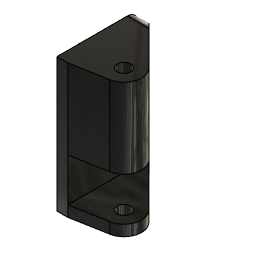
3030 Idler Bracket B Front_1X v4 (Autodesk Fusion 360 design; units mm, degrees)
Autodesk Fusion 360 part; units mm, degrees
sketch "Sketch1" plane through (0, 0, 0) normal (1, 0, 0) x (0, 1, 0)
  line L0 (0, 16) -> (20, 16)
  line L1 (20, 16) -> (20, 0)
  line L2 (20, 0) -> (0, 0)
  line L3 (0, 0) -> (0, 16)
  dimension "d2462_1" = 20
  dimension "d2463_1" = 16
  constraint horizontal L0
  constraint vertical L1
  constraint horizontal L2
  constraint vertical L3
  constraint coincident L2.end L3.start
  measures "d2462_1" distance of L0.start L0.end
  measures "d2463_1" distance of L0.start L2.end
extrude "Extrude1" add sketch "Sketch1" along normal blind 4
sketch "Sketch2" plane through (0, 0, 16) normal (0, 0, 1) x (-1, 0, 0)
  line L0 (0, -20) -> (0, 0)
  line L1 (0, 0) -> (-4, 0)
  line L2 (-4, 0) -> (-4, -20)
  line L3 (-4, -20) -> (0, -20)
  line L4 (-4, -10) -> (-29.8619, -10) construction
  circle A0 centre (-16, -21.24) radius 6 construction
  circle A1 centre (-42.1729, -8.5) radius 6.11 construction
  line L5 (-16, -15.24) -> (-27.2824, -15.24) construction
  line L6 (-42.1729, -14.61) -> (-27.2824, -14.61) construction
  line L7 (-27.2824, -15.24) -> (-27.2824, -14.61) construction
  line L8 (-16, -15.24) -> (-16, -13.84) construction
  line L9 (-16, -13.84) -> (-48.5157, -13.84) construction
  circle A2 centre (-16, -21.24) radius 2.5
  arc A3 (-20.6028, -16.6504) -> (-11.9535, -26.3269) centre (-16, -21.24) ccw
  line L10 (-4, -20) -> (-11.9535, -26.3269)
  line L11 (-4, 0) -> (-20.6028, -16.6504)
  dimension "d4861_1" = 12
  dimension "d4864_1" = 12
  dimension "d4867_1" = 12.22
  dimension "d4871_1" = 0.63
  dimension "d4872_1" = 1.4
  dimension "d4873_1" = 0.77
  dimension "d4874_1" = 5
  dimension "d4876_1" = 4
  dimension "d5002" = 8.5
  constraint midpoint L2 L4.start
  constraint perpendicular L2 L4
  constraint coincident A0 L5.start
  constraint tangent A0 L5
  constraint parallel L4 L5
  constraint coincident A1 L6.start
  constraint horizontal L6
  constraint perpendicular L5 L7
  constraint coincident L6.end L7.end
  constraint tangent A1 L6
  constraint perpendicular L5 L8
  constraint perpendicular L8 L9
  constraint concentric A0 A2
  constraint concentric A2 A3
  constraint coincident L2.end L3.start
  constraint coincident L1.end L2.start
  constraint tangent A3 L10
  constraint tangent A3 L11
  measures "d4861_1" diameter of A0
  measures "d4864_1" distance of L2 A0.centre
  measures "d4867_1" diameter of A1
  measures "d4871_1" distance of L5.end L6.end
  measures "d4872_1" distance of L5 L9
  measures "d4873_1" distance of A1 L9
  measures "d4874_1" diameter of A2
  measures "d4876_1" distance of A2 A3
  measures "d5002" distance of L1 A1.centre
extrude "Extrude2" add sketch "Sketch2" along normal blind 4
extrude "Extrude3" add sketch "Sketch2" against normal blind 4 from surface at -16
extrude "Extrude6" add 1 faces at (1.3333, 20, 10.6667) along direction (0, 1, 0) blind 10
sketch "Sketch5" plane through (0, 0, 20) normal (0, 0, 1) x (-1, 0, 0)
  line L0 (0, -30) -> (0, 0)
  line L1 (0, 0) -> (-4, 0)
  line L2 (-4, -20) -> (-4, -30)
  line L3 (-4, -30) -> (0, -30)
  line L4 (-4, -30) -> (0, -30)
  line L5 (0, 0) -> (0, -30)
  line L6 (-4, -20) -> (-4, -30)
  line L7 (-4, 0) -> (0, 0)
  line L8 (-4, -30) -> (-17.1494, -27.6376)
  circle A0 centre (-16, -21.24) radius 2.5
  line L9 (-4, 0) -> (-20.6028, -16.6504)
  arc A1 (-20.6028, -16.6504) -> (-11.9535, -26.3269) centre (-16, -21.24) ccw
  line L10 (-11.9535, -26.3269) -> (-4, -20)
  circle A2 centre (-16, -21.24) radius 2.5
  line L11 (-20.6028, -16.6504) -> (-4, 0)
  arc A3 (-20.6028, -16.6504) -> (-11.9535, -26.3269) centre (-16, -21.24) ccw
  line L12 (-4, -20) -> (-11.9535, -26.3269)
  constraint coincident L6 L2.end
  constraint coincident L8.end A3
  constraint tangent L8 A3
  constraint coincident L2.end L3.start
extrude "Extrude7" add sketch "Sketch5" against normal up to surface (4 mm away) contours L2 L6 L8 A1 L10 A3 L12
extrude "Extrude8" add sketch "Sketch5" along normal up to surface (4 mm away) from surface at -24 contours L2 L6 L8 A1 L10 A3 L12
sketch "Sketch4" plane through (4, 0, 0) normal (1, 0, 0) x (0, 1, 0)
  line L0 (0, 0) -> (30, 0)
  line L1 (30, 16) -> (0, 16)
  line L2 (30, -4) -> (0, -4)
  line L3 (0, 20) -> (30, 20)
  line L4 (0, 8) -> (10, 8)
  line L5 (30, 8) -> (15, 8)
  line L6 (30, 0) -> (30, 16)
  line L7 (0, 16) -> (0, 0)
  line L8 (0, -4) -> (0, 20)
  line L9 (30, 20) -> (30, -4)
  dimension "d14_3_1" = 10
  dimension "d15_3_1" = 15
  constraint midpoint L5.start L9
  constraint midpoint L4.start L8
  constraint horizontal L4
  constraint horizontal L5
  measures "d14_3_1" distance of L4.start L4.end
  measures "d15_3_1" distance of L5.start L5.end
hole "Hole1" at (4, 15, 8) direction (-1, 0, 0) diameter 5.5 depth 28.1 tip angle 118
sketch "Sketch6" plane through (0, 0, -4) normal (0, 0, -1) x (-1, 0, 0)
  line L0 (0, 20) -> (-45, 20)
  line L1 (-45, 20) -> (-45, 0)
  line L2 (-45, 0) -> (0, 0)
  line L3 (0, 0) -> (0, 20)
  circle A0 centre (-16, 21.24) radius 2.5
  line L4 (0, 0) -> (0, 30)
  line L5 (0, 30) -> (-4, 30)
  line L6 (-4, 30) -> (-17.1494, 27.6376)
  arc A1 (-17.1494, 27.6376) -> (-20.6028, 16.6504) centre (-16, 21.24) ccw
  line L7 (-20.6028, 16.6504) -> (-4, 0)
  line L8 (-4, 0) -> (0, 0)
  dimension "d4947_1" = 45
  dimension "d4948_1" = 20
  constraint horizontal L0
  constraint vertical L1
  constraint horizontal L2
  constraint vertical L3
  constraint coincident L2.end L3.start
  measures "d4947_1" distance of L0.start L0.end
  measures "d4948_1" distance of L0.start L2.end
extrude "Extrude9" add sketch "Sketch6" along normal blind 25.5 contours L0 L2 L3 A0 L4 A1 L7 L8 | L0 A0 L4 L5 L6 A1
fillet "Fillet2" radius 4 2 edges at (2, 0, -29.5) (2, 0, 20)
move_body "Move1" bodies 1 to x (1, 0, 0) y (0, -1, 0) z (0, 0, -1) at (0, 42.48, 0)
equation "d2463_1 = idler_height_gates + 2 * idler_shim_thickness"
equation "d2464_1 = Part_Thickness_3"
equation "d2476_1 = Part_Thickness"
equation "d2479_1 = -Part_Thickness"
equation "d4861_1 = idler_smooth_od"
equation "d4867_1 = Pulley_od"
equation "d4872_1 = belt_thickness"
equation "d4949_1 = 2 * idler_height_gates - idler_gates_flange_thickness - idler_shim_thickness"
equation "d5002 = idler_offset"
equation "Part_Thickness = 4 mm" comment "Thickness of Printed Parts"
equation "belt_thickness = 1.4 mm" comment "Thickness of GT2 9mm Belt"
equation "idler_smooth_gates_od = 12 mm" comment "Idler Outer Diameter"
equation "Pulley_od = 12.22 mm" comment "GT2 Pulley/Idler Tooth OD"
equation "idler_height_gates = 14 mm" comment "Gates 2GT Idler Height"
equation "idler_shim_thickness = 1 mm" comment "Shim Idler Thickness"
equation "idler_gates_flange_thickness = 1.5 mm" comment "Gates Idler Pulley Flange Thickness"
equation "idler_smooth_od = idler_smooth_gates_od" comment "Choose your idler smooth OD"
equation "Part_Thickness_3 = 4 mm" comment "Thickness of Printed Parts"
equation "idler_offset = 8.5 mm" comment "Idler offset"
named bodies: "AB Idler Bracket Front"
